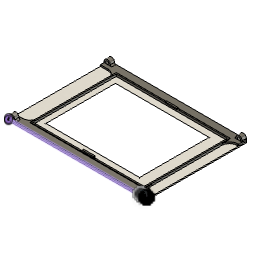
Inkplate 6 PCB Holder 130x180 mm Photo Frame v1 (Autodesk Fusion 360 design; units mm, degrees)
Autodesk Fusion 360 part; units mm, degrees
sketch "Sketch1" plane through (0, 0, 0) normal (0, 1, 0) x (1, 0, 0)
  line L0 (-90, -65) -> (90, -65)
  line L1 (90, -65) -> (90, 65)
  line L2 (90, 65) -> (-90, 65)
  line L3 (-90, 65) -> (-90, -65)
  line L4 (-90, -65) -> (90, 65) construction
  line L5 (90, -65) -> (-90, 65) construction
  line L6 (-61, -45.3) -> (61, -45.3)
  line L7 (61, -45.3) -> (61, 45.3)
  line L8 (61, 45.3) -> (-61, 45.3)
  line L9 (-61, 45.3) -> (-61, -45.3)
  line L10 (-61, -45.3) -> (61, 45.3) construction
  line L11 (61, -45.3) -> (-61, 45.3) construction
  line L12 (76.5, -45.3) -> (76.5, 45.3) construction
  line L13 (61, 53.3) -> (-61, 53.3) construction
  line L14 (-61, -54.8) -> (61, -54.8) construction
  line L15 (-68, 45.3) -> (-68, -45.3) construction
  line L16 (-68, 53.3) -> (76.5, 53.3)
  line L17 (76.5, 53.3) -> (76.5, -54.8)
  line L18 (76.5, -54.8) -> (-68, -54.8)
  line L19 (-68, -54.8) -> (-68, 53.3)
  line L20 (32.0539, 9.3491) -> (-36.4423, 9.3491) construction
  line L21 (-36.4423, 9.3491) -> (-36.4423, 14.8822) construction
  line L22 (-36.4423, 14.8822) -> (32.0539, 14.8822) construction
  line L23 (32.0539, 14.8822) -> (32.0539, 9.3491) construction
  dimension "d1" = 180
  dimension "d2" = 130
  dimension "d3" = 122
  dimension "d4" = 90.6
  dimension "d9" = 10
  dimension "d12" = 108.1
  dimension "d13" = 144.5
  constraint perpendicular L0 L1
  constraint parallel L0 L2
  constraint parallel L1 L3
  constraint coincident L4 origin
  constraint coincident L5 origin
  constraint perpendicular L6 L7
  constraint parallel L6 L8
  constraint parallel L7 L9
  constraint coincident L10 origin
  constraint coincident L11 origin
  constraint collinear L14 L18
  constraint collinear L13 L16
  constraint collinear L15 L19
  constraint collinear L12 L17
  measures "d1" distance of L1.end L2.end
  measures "d2" distance of L0.end L1.end
  measures "d3" distance of L7.end L8.end
  measures "d4" distance of L6.end L7.end
  measures "d12" distance of L16.start L18.end
  measures "d13" distance of L16.start L16.end
extrude "Extrude5" add sketch "Sketch1" along normal blind 1.5 contours L0 L1 L2 L3 | L16 L17 L18 L19 makes body 1
sketch "Sketch8" plane through (0, 1.5, 0) normal (0, 1, 0) x (-1, 0, 0)
  line L0 (61, 45.3) -> (61, -45.3)
  line L1 (61, -45.3) -> (-61, -45.3)
  line L2 (-61, -45.3) -> (-61, 45.3)
  line L3 (-61, 45.3) -> (61, 45.3)
  line L4 (90, -65) -> (90, 65)
  line L5 (90, 65) -> (-90, 65)
  line L6 (-90, 65) -> (-90, -65)
  line L7 (-90, -65) -> (90, -65)
  line L8 (68, 54.8) -> (68, -53.3)
  line L9 (-76.5, 54.8) -> (68, 54.8)
  line L10 (-61, 45.3) -> (-61, -45.3)
  line L11 (-61, -45.3) -> (61, -45.3)
  line L12 (61, -45.3) -> (61, 45.3)
  line L13 (61, 45.3) -> (-61, 45.3)
  line L14 (-76.5, -53.3) -> (-76.5, 54.8)
  line L15 (68, -53.3) -> (-76.5, -53.3)
  line L16 (-76.8, -53.6) -> (-76.8, 55.1)
  line L17 (-76.8, 55.1) -> (68.3, 55.1)
  line L18 (68.3, 55.1) -> (68.3, -53.6)
  line L19 (68.3, -53.6) -> (-76.8, -53.6)
  line L20 (-78.47, -55.27) -> (-78.47, 56.77)
  line L21 (-78.47, 56.77) -> (69.97, 56.77)
  line L22 (69.97, 56.77) -> (69.97, -55.27)
  line L23 (69.97, -55.27) -> (-78.47, -55.27)
  dimension "PCBToleranceOffset" = -0.3
extrude "Extrude1" add sketch "Sketch8" along normal blind 2.8 separate body contours L20 L21 L22 L23 makes body 2 in component "pcbHolder"
chamfer "Chamfer2" distance 1.5 angle 45 4 edges at (0, 0, 45.3) (-61, 0, 0) (61, 0, 0) (0, 0, -45.3) on bodies 1
sketch "Sketch9" plane through (0, 0, 65) normal (0, 0, 1) x (1, 0, 0)
  line L0 (-90, 0) -> (90, 0)
  line L1 (90, 0) -> (90, 1.5)
  line L2 (90, 1.5) -> (-90, 1.5)
  line L3 (-90, 1.5) -> (-90, 0)
  line L4 (-69.97, 1.5) -> (78.47, 1.5)
  line L5 (78.47, 1.5) -> (78.47, 4.3)
  line L6 (78.47, 4.3) -> (-69.97, 4.3)
  line L7 (-69.97, 4.3) -> (-69.97, 1.5)
  line L8 (78.47, 1.5) -> (90, 1.5) construction
  line L9 (84.235, 1.5) -> (84.235, 3.45) construction
  circle A0 centre (84.2347, 5.1) radius 1.65
  dimension "d145" = 1.95
  dimension "d146" = 3.3
  dimension "d147" = 3.45
  constraint coincident L4.end L5.start
  constraint coincident L1.end L2.start
  constraint midpoint L8 L9.start
  constraint perpendicular L2 L9
  constraint coincident L9.end A0
  measures "d145" distance of L9.start L9.end
  measures "d146" diameter of A0
  measures "d147" distance of L0 L9.end
sketch "Sketch1 (2)" plane through (0, 1.5, 0) normal (0, 1, 0) x (-1, 0, 0) in component "pcbHolder"
  line L0 (61, 45.3) -> (61, -45.3)
  line L1 (61, -45.3) -> (-61, -45.3)
  line L2 (-61, -45.3) -> (-61, 45.3)
  line L3 (-61, 45.3) -> (61, 45.3)
  line L4 (90, -65) -> (90, 65)
  line L5 (90, 65) -> (-90, 65)
  line L6 (-90, 65) -> (-90, -65)
  line L7 (-90, -65) -> (90, -65)
  line L8 (68.3, 55.1) -> (68.3, -53.6)
  line L9 (68.3, -53.6) -> (-76.8, -53.6)
  line L10 (-76.8, -53.6) -> (-76.8, 55.1)
  line L11 (-76.8, 55.1) -> (68.3, 55.1)
  line L12 (69.97, -55.27) -> (69.97, 56.77)
  line L13 (69.97, 56.77) -> (-78.47, 56.77)
  line L14 (-78.47, 56.77) -> (-78.47, -55.27)
  line L15 (-78.47, -55.27) -> (69.97, -55.27)
  line L16 (-78.47, 56.77) -> (-90, 56.77)
  line L17 (-90, 56.77) -> (90, 56.77)
  line L18 (90, -54.6) -> (-90, -54.6)
  constraint coincident L13.end L14.start
  constraint coincident L6 L16.end
  constraint perpendicular L6 L16
  constraint coincident L4 L17.end
  constraint perpendicular L4 L17
  constraint coincident L4 L18.start
  constraint coincident L6 L18.end
  constraint perpendicular L6 L18
extrude "Extrude2" add sketch "Sketch1 (2)" along normal blind 1.95 contours L4 L6 L7 L12 L14 L15 L18 | L4 L5 L6 L13 L16 L17 | L12 L14 L15 L18 bodies 2 in component "pcbHolder"
sketch "Sketch2" plane through (0, 1.5, 0) normal (0, 1, 0) x (-1, 0, 0) in component "pcbHolder"
  line L0 (61, 45.3) -> (61, -45.3)
  line L1 (61, -45.3) -> (-61, -45.3)
  line L2 (-61, -45.3) -> (-61, 45.3)
  line L3 (-61, 45.3) -> (61, 45.3)
  line L4 (90, -65) -> (90, 65)
  line L5 (90, 65) -> (-90, 65)
  line L6 (-90, 65) -> (-90, -65)
  line L7 (-90, -65) -> (90, -65)
  line L8 (90, -54.6) -> (69.97, -54.6)
  line L9 (90, -65) -> (90, -54.6)
  line L10 (-90, -65) -> (90, -65)
  line L11 (-90, -54.6) -> (-90, -65)
  line L12 (-78.47, -54.6) -> (-90, -54.6)
  line L13 (69.97, 56.77) -> (90, 56.77)
  line L14 (-90, 65) -> (-90, 56.77)
  line L15 (90, 65) -> (-90, 65)
  line L16 (90, 56.77) -> (90, 65)
  line L17 (-90, 56.77) -> (-78.47, 56.77)
  line L18 (-76.8, 55.1) -> (68.3, 55.1)
  line L19 (-76.8, -53.6) -> (-76.8, 55.1)
  line L20 (68.3, -53.6) -> (-76.8, -53.6)
  line L21 (68.3, 55.1) -> (68.3, -53.6)
  line L22 (-78.47, -54.6) -> (-78.47, 56.77)
  line L23 (69.97, 56.77) -> (69.97, -54.6)
  circle A0 centre (79.97, -44.6) radius 10
  circle A1 centre (-88.47, -44.6) radius 10
  circle A2 centre (79.97, 46.77) radius 10
  circle A3 centre (-88.47, 46.77) radius 10
  dimension "d150" = 10
  dimension "d151" = 10
  dimension "d152" = 10
  dimension "d153" = 10
  constraint tangent L8 A0
  constraint tangent L23 A0
  constraint tangent L12 A1
  constraint tangent L22 A1
  constraint tangent L23 A2
  constraint tangent L13 A2
  constraint tangent L17 A3
  constraint tangent L22 A3
  measures "d150" radius of A0
  measures "d151" radius of A1
  measures "d152" radius of A2
  measures "d153" radius of A3
extrude "Extrude3" add sketch "Sketch2" along normal up to surface (1.95 mm away) contours L8 L23 A0 | L13 L23 A2 | L12 L22 A1 | L17 L22 A3 bodies 2 in component "pcbHolder"
sketch "Sketch3" plane through (0, 4.3, 0) normal (0, 1, 0) x (-1, 0, 0) in component "pcbHolder"
  line L0 (68.3, 55.1) -> (68.3, -53.6)
  line L1 (68.3, -53.6) -> (-76.8, -53.6)
  line L2 (-76.8, -53.6) -> (-76.8, 55.1)
  line L3 (-76.8, 55.1) -> (68.3, 55.1)
  line L4 (69.97, -55.27) -> (69.97, 56.77)
  line L5 (69.97, 56.77) -> (-78.47, 56.77)
  line L6 (-78.47, 56.77) -> (-78.47, -55.27)
  line L7 (-78.47, -55.27) -> (69.97, -55.27)
  line L8 (-4.25, 55.1) -> (-4.25, -53.6) construction
  line L9 (-11.75, 56.1) -> (3.25, 56.1)
  line L10 (3.25, 56.1) -> (3.25, 54.1)
  line L11 (3.25, 54.1) -> (-11.75, 54.1)
  line L12 (-11.75, 54.1) -> (-11.75, 56.1)
  line L13 (-11.75, 56.1) -> (3.25, 54.1) construction
  line L14 (3.25, 56.1) -> (-11.75, 54.1) construction
  point P0 (-4.25, 55.1)
  dimension "d156" = 15
  constraint midpoint L3 P0
  constraint midpoint L1 L8.end
  constraint horizontal L9
  constraint perpendicular L9 L10
  constraint parallel L9 L11
  constraint parallel L10 L12
  constraint coincident L13 P0
  constraint coincident L14 P0
  constraint coincident P0 L8.start
  measures "d156" distance of L10.end L11.end
extrude "Extrude4" add sketch "Sketch3" along normal blind 1.5 contours L3 L10 L11 L12 | L3 L9 L10 L12 bodies 2 in component "pcbHolder"
fillet "Fillet1" radius 2 2 edges at (-3.25, 4.3, 55.6) (11.75, 4.3, 55.6) on bodies 2 in component "pcbHolder"
ref_plane "WorkPlane1" through (4.25, 2.9, 0.75) normal (0, 0, 1) x (1, 0, 0) in component "pcbHolder"
mirror "Mirror1" about plane through (4.25, 2.9, 0.75) normal (0, 0, 1) of "Extrude4", "Fillet1" in component "pcbHolder"
sketch "Sketch5" plane through (0, 0, 65) normal (0, 0, 1) x (1, 0, 0) in component "pcbHolder"
  line L0 (-90, 1.5) -> (90, 1.5)
  line L1 (90, 1.5) -> (90, 3.45)
  line L2 (90, 3.45) -> (-90, 3.45)
  line L3 (-90, 3.45) -> (-90, 1.5)
  line L4 (90, 3.45) -> (86, 3.45) construction
  line L5 (-90, 0) -> (90, 0)
  line L6 (90, 0) -> (90, 1.5)
  line L7 (90, 1.5) -> (-90, 1.5)
  line L8 (-90, 1.5) -> (-90, 0)
  circle A0 centre (86, 5.1) radius 2
  circle A1 centre (86, 5.1) radius 4
  line L9 (89.9983, 4.9837) -> (90, 3.45)
  line L10 (82.0021, 4.9715) -> (82.0021, 3.45)
  dimension "d163" = 4
  dimension "d164" = 1.95
  dimension "ScrewDiameter" = 4
  dimension "d166" = 2
  constraint coincident L1.end L2.start
  constraint perpendicular L1 L4
  constraint coincident A1 L9.start
  constraint coincident A1 L10.start
  constraint coincident L2 L10.end
  constraint perpendicular L2 L10
  measures "d163" distance of L1.end L4.end
  measures "d164" distance of L0.end L1.end
  measures "ScrewDiameter" diameter of A0
  measures "d166" distance of A0
extrude "Extrude5'" add sketch "Sketch5" against normal blind 5.5 contours L2 A0 A1 | L2 A1 L10 | L2 A1 L9 bodies 2 in component "pcbHolder"
mirror "Mirror2" about plane through (0, 0, 0) normal (1, 0, 0) of "Extrude5'" in component "pcbHolder"
mirror "Mirror3" about plane through (0, 0, 0) normal (0, 0, 1) of "Extrude5'", "Mirror2" in component "pcbHolder"
fillet "Fillet2" radius 2 4 edges at (-82.0021, 3.45, -62.25) (-82.0021, 3.45, 62.25) (82.0021, 3.45, 62.25) (82.0021, 3.45, -62.25) on bodies 2 in component "pcbHolder"
extrude "Extrude6" cut sketch "Sketch5" against normal up to surface (5.5 mm away) contours L2 A0 picked at (86.3002, 3.4048) bodies 2 in component "pcbHolder"
mirror "Mirror4" about plane through (0, 0, 0) normal (1, 0, 0) of "Extrude6" in component "pcbHolder"
mirror "Mirror5" about plane through (0, 0, 0) normal (0, 0, 1) of "Extrude6", "Mirror4" in component "pcbHolder"
sketch "Sketch4" plane through (0, 0, 65) normal (0, 0, 1) x (1, 0, 0) in component "pcbHolder"
  arc A0 (11.75, 5.8) -> (13.6865, 4.3) centre (13.6865, 6.3) ccw
  arc A1 (-5.1865, 4.3) -> (-3.25, 5.8) centre (-5.1865, 6.3) ccw
  line L0 (-3.25, 5.8) -> (11.75, 5.8)
  line L1 (77.8, 4.3) -> (13.6865, 4.3)
  line L2 (-5.1865, 4.3) -> (-69.3, 4.3)
  line L3 (77.8, 3.45) -> (77.8, 4.3)
  line L4 (-69.3, 3.45) -> (-69.3, 4.3)
  line L5 (-90, 1.5) -> (-90, 3.45)
  line L6 (90, 1.5) -> (-90, 1.5)
  line L7 (90, 3.45) -> (77.8, 3.45)
  line L8 (-69.3, 3.45) -> (-90, 3.45)
  line L9 (90, 1.5) -> (90, 3.45)
extrude "Extrude1'" [suppressed]
extrude "Extrude2'" [suppressed]
chamfer "Chamfer1" [suppressed]
sketch "Sketch2 (2)" plane through (0, 3.3, 0) normal (0, 1, 0) x (-1, 0, 0)
  line L0 (-76.5, 54.8) -> (68, 54.8)
  line L1 (68, 54.8) -> (68, -53.3)
  line L2 (68, -53.3) -> (-76.5, -53.3)
  line L3 (-76.5, -53.3) -> (-76.5, 54.8)
  line L4 (90, -65) -> (90, 65)
  line L5 (90, 65) -> (-90, 65)
  line L6 (-90, 65) -> (-90, -65)
  line L7 (-90, -65) -> (90, -65)
  line L8 (-78, -54.8) -> (-78, 56.3)
  line L9 (-78, 56.3) -> (69.5, 56.3)
  line L10 (69.5, 56.3) -> (69.5, -54.8)
  line L11 (69.5, -54.8) -> (-78, -54.8)
  dimension "d20" = -1.5
extrude "Extrude3'" [suppressed]
sketch "Sketch3 (2)" plane through (0, 3.3, 0) normal (0, 1, 0) x (-1, 0, 0)
  line L0 (69.5, -54.8) -> (-78, -54.8)
  line L1 (-78, -54.8) -> (-78, 56.3)
  line L2 (-78, 56.3) -> (69.5, 56.3)
  line L3 (69.5, 56.3) -> (69.5, -54.8)
  line L4 (90, -65) -> (90, 65)
  line L5 (90, 65) -> (-90, 65)
  line L6 (-90, 65) -> (-90, -65)
  line L7 (-90, -65) -> (90, -65)
copy_body "Body->Comp1" [suppressed] in component "Component"
ref_plane "WorkPlane2" through (0, 1.65, 62) normal (0, 0, 1) x (1, 0, 0)
sketch "Sketch4 (2)" plane through (0, 0, 62) normal (0, 0, 1) x (1, 0, 0)
  line L0 (-90, 0) -> (90, 0)
  line L1 (90, 0) -> (90, 3.3)
  line L2 (90, 3.3) -> (-90, 3.3)
  line L3 (-90, 3.3) -> (-90, 0)
  line L4 (-68, 0.55) -> (76.5, 0.55)
  line L5 (76.5, 0.55) -> (76.5, 4.3)
  line L6 (76.5, 4.3) -> (-68, 4.3)
  line L7 (-68, 4.3) -> (-68, 0.55)
  line L8 (82.5, -5.45) -> (82.5, 10.3) construction
  line L9 (82.5, 10.3) -> (-74, 10.3) construction
  line L10 (-74, 10.3) -> (-74, -5.45) construction
  line L11 (-74, -5.45) -> (82.5, -5.45) construction
  line L12 (-74, 3.3) -> (-74, 5.1) construction
  circle A0 centre (-74, 5.1) radius 1.65
  line L13 (4.25, -5.45) -> (4.25, 10.3)
  circle A1 centre (-74, 5.1) radius 4
  circle A2 centre (82.5, 5.1) radius 4
  dimension "d85" = 6
  dimension "d86" = 1.8
  dimension "d87" = 3.3
  dimension "d88" = 8
  constraint coincident L10 L12.start
  constraint coincident L2 L12.start
  constraint perpendicular L2 L12
  constraint coincident L12.end A0.centre
  constraint midpoint L11 L13.start
  constraint midpoint L9 L13.end
  constraint symmetric L13 A1 A2
  measures "d86" distance of L12.start L12.end
  measures "d87" diameter of A0
  measures "d88" diameter of A1
extrude "Extrude4'" [suppressed]
extrude "Extrude8" [no effect] in component "Component"
ref_plane "WorkPlane3" through (0, 1.65, 0) normal (0, 0, -1) x (-1, 0, 0)
mirror "Mirror1'" [suppressed]
mirror "Mirror1''" [no effect] in component "Component"
sketch "Sketch5 (2)" plane through (0, 3.3, 0) normal (0, 1, 0) x (-1, 0, 0)
  line L0 (70.4279, -62) -> (70.4279, -37)
  line L1 (70.4279, -37) -> (77.5721, -37)
  line L2 (77.5721, -37) -> (77.5721, -62)
  line L3 (77.5721, -62) -> (70.4279, -62)
  line L4 (-86.0721, -62) -> (-86.0721, -37)
  line L5 (-86.0721, -37) -> (-78.9279, -37)
  line L6 (-78.9279, -37) -> (-78.9279, -62)
  line L7 (-78.9279, -62) -> (-86.0721, -62)
  line L8 (70.4279, 37) -> (70.4279, 62)
  line L9 (70.4279, 62) -> (77.5721, 62)
  line L10 (77.5721, 62) -> (77.5721, 37)
  line L11 (77.5721, 37) -> (70.4279, 37)
  line L12 (-86.0721, 37) -> (-86.0721, 62)
  line L13 (-86.0721, 62) -> (-78.9279, 62)
  line L14 (-78.9279, 62) -> (-78.9279, 37)
  line L15 (-78.9279, 37) -> (-86.0721, 37)
  line L16 (69.5, -54.8) -> (-78, -54.8)
  line L17 (-78, -54.8) -> (-78, 56.3)
  line L18 (-78, 56.3) -> (69.5, 56.3)
  line L19 (69.5, 56.3) -> (69.5, -54.8)
  line L20 (90, -65) -> (90, 65)
  line L21 (90, 65) -> (-90, 65)
  line L22 (-90, 65) -> (-90, -65)
  line L23 (-90, -65) -> (90, -65)
  line L24 (-90, 0) -> (90, 0)
  line L25 (88, 63) -> (-88, 63) construction
  line L26 (-88, 63) -> (-88, -63) construction
  line L27 (-88, -63) -> (88, -63) construction
  line L28 (88, -63) -> (88, 63) construction
  line L29 (85.5, 60.5) -> (-85.5, 60.5) construction
  line L30 (-85.5, 60.5) -> (-85.5, -60.5) construction
  line L31 (-85.5, -60.5) -> (85.5, -60.5) construction
  line L32 (85.5, -60.5) -> (85.5, 60.5) construction
  line L33 (83.5, 58.5) -> (-83.5, 58.5)
  line L34 (-83.5, 58.5) -> (-83.5, -58.5)
  line L35 (-83.5, -58.5) -> (83.5, -58.5)
  line L36 (83.5, -58.5) -> (83.5, 58.5)
  line L37 (77.5721, -60.5) -> (70.4279, -60.5)
  line L38 (70.4279, -60.5) -> (70.4279, -65)
  line L39 (70.4279, -65) -> (77.5721, -65)
  line L40 (77.5721, -65) -> (77.5721, -60.5)
  line L41 (77.5721, -58.5) -> (70.4279, -58.5)
  line L42 (70.4279, -58.5) -> (70.4279, -60.5)
  line L43 (70.4279, -60.5) -> (77.5721, -60.5)
  line L44 (77.5721, -60.5) -> (77.5721, -58.5)
  line L45 (77.5721, -62) -> (70.4279, -62)
  line L46 (70.4279, -62) -> (70.4279, -60.5)
  line L47 (70.4279, -60.5) -> (77.5721, -60.5)
  line L48 (77.5721, -60.5) -> (77.5721, -62)
  line L49 (70.4279, -58.5) -> (68.4279, -58.5) construction
  line L50 (68.4279, -58.5) -> (70.4279, -58.5)
  line L51 (70.4279, -58.5) -> (70.4279, -65)
  line L52 (70.4279, -65) -> (68.4279, -65)
  line L53 (68.4279, -65) -> (68.4279, -58.5)
  line L54 (74, -65) -> (74, -37)
  line L55 (79.5721, -65) -> (79.5721, -58.5)
  line L56 (77.5721, -63) -> (70.4279, -63)
  line L57 (70.4279, -63) -> (70.4279, -60.5)
  line L58 (70.4279, -60.5) -> (77.5721, -60.5)
  line L59 (77.5721, -60.5) -> (77.5721, -63)
  dimension "d99" = -2
  dimension "d101" = -4.5
  dimension "d102" = -6.5
  dimension "d103" = 2
  dimension "d136" = 7.1442
  constraint midpoint L22 L24.start
  constraint midpoint L20 L24.end
  constraint horizontal L37
  constraint vertical L38
  constraint horizontal L39
  constraint vertical L40
  constraint coincident L23 L38.end
  constraint coincident L2 L37.start
  constraint coincident L31 L37.start
  constraint horizontal L41
  constraint vertical L42
  constraint horizontal L43
  constraint vertical L44
  constraint coincident L2 L41.start
  constraint coincident L35 L41.start
  constraint horizontal L45
  constraint vertical L46
  constraint horizontal L47
  constraint vertical L48
  constraint coincident L2.end L3.start
  constraint collinear L0 L38
  constraint perpendicular L42 L49
  constraint horizontal L50
  constraint vertical L51
  constraint horizontal L52
  constraint vertical L53
  constraint midpoint L39 L54.start
  constraint midpoint L1 L54.end
  constraint symmetric L49.end L54 L55.end
  constraint symmetric L52.end L54 L55.start
  constraint horizontal L56
  constraint vertical L57
  constraint horizontal L58
  constraint vertical L59
  constraint coincident L40 L56.start
  constraint coincident L27 L56.start
  measures "d103" distance of L41.end L49.end
  measures "d136" distance of L2.end L0.start
extrude "Extrude9" [suppressed] in component "Component"
fillet "Fillet1'" [suppressed] in component "Component"
ref_plane "WorkPlane4" through (4.25, 3.8, 0.75) normal (-1, 0, 0) x (0, 0, 1)
mirror "Mirror2'" [suppressed] in component "Component"
mirror "Mirror3'" [suppressed] in component "Component"
mirror "Mirror4'" [suppressed] in component "Component"
fillet "Fillet2'" [suppressed] in component "Component"
fillet "Fillet3" [suppressed] in component "Component"
extrude "Extrude12" [suppressed] in component "Component"
fillet "Fillet4" [suppressed] in component "Component"
extrude "Extrude10" [suppressed] in component "Component"
mirror "Mirror5'" [suppressed] in component "Component"
sketch "Sketch6" plane through (0, 8.3, 0) normal (0, 1, 0) x (-1, 0, 0)
  line L0 (70.4279, -63) -> (70.4279, -60.5)
  line L1 (70.4279, -60.5) -> (77.5721, -60.5)
  line L2 (77.5721, -60.5) -> (77.5721, -63)
  line L3 (69.928, -65) -> (78.072, -65)
  line L4 (78.072, -58.5) -> (69.928, -58.5)
  line L5 (70.4279, 60.5) -> (70.4279, 63)
  line L6 (77.5721, 63) -> (77.5721, 60.5)
  line L7 (77.5721, 60.5) -> (70.4279, 60.5)
  line L8 (78.072, 65) -> (69.928, 65)
  line L9 (69.928, 58.5) -> (78.072, 58.5)
  line L10 (-78.9279, -60.5) -> (-78.9279, -63)
  line L11 (-86.0721, -63) -> (-86.0721, -60.5)
  line L12 (-86.0721, -60.5) -> (-78.9279, -60.5)
  line L13 (-88, -65) -> (-76.9279, -65)
  line L14 (-76.9279, -58.5) -> (-90, -58.5)
  line L15 (-78.9279, 63) -> (-78.9279, 60.5)
  line L16 (-78.9279, 60.5) -> (-86.0721, 60.5)
  line L17 (-86.0721, 60.5) -> (-86.0721, 63)
  line L18 (-76.9279, 65) -> (-88, 65)
  line L19 (-90, 58.5) -> (-76.9279, 58.5)
  line L20 (77.5721, -63) -> (70.4279, -63)
  line L21 (70.4279, 63) -> (77.5721, 63)
  line L22 (-78.9279, -63) -> (-86.0721, -63)
  line L23 (-86.0721, 63) -> (-78.9279, 63)
  line L24 (78.072, -65) -> (78.072, -58.5)
  line L25 (69.928, -58.5) -> (69.928, -65)
  line L26 (78.072, 58.5) -> (78.072, 65)
  line L27 (69.928, 65) -> (69.928, 58.5)
  arc A0 (-90, -63) -> (-88, -65) centre (-88, -63) ccw
  line L28 (-76.9279, -65) -> (-76.9279, -58.5)
  line L29 (-90, -58.5) -> (-90, -63)
  arc A1 (-88, 65) -> (-90, 63) centre (-88, 63) ccw
  line L30 (-90, 63) -> (-90, 58.5)
  line L31 (-76.9279, 58.5) -> (-76.9279, 65)
extrude "Extrude11" [suppressed] in component "Component"
fillet "Fillet5" [suppressed] in component "Component"
ref_plane "WorkPlane5" through (0, 1.5, 0) normal (0, -1, 0) x (-1, 0, 0)
split "Split1" [suppressed] in component "Component"
sketch "Sketch7" plane through (0, 3.3, 0) normal (0, 1, 0) x (-1, 0, 0)
  arc A0 (88, -65) -> (90, -63) centre (88, -63) ccw
  line L0 (90, -63) -> (90, 63)
  arc A1 (90, 63) -> (88, 65) centre (88, 63) ccw
  line L1 (88, 65) -> (85.4882, 65)
  line L2 (85.4882, 65) -> (85.4882, 58.5)
  line L3 (85.4882, 58.5) -> (77.5721, 58.5)
  line L4 (77.5721, 58.5) -> (77.5721, 37)
  line L5 (77.5721, 37) -> (70.4279, 37)
  line L6 (70.4279, 37) -> (70.4279, 58.5)
  line L7 (70.4279, 58.5) -> (62.5118, 58.5)
  line L8 (62.5118, 58.5) -> (62.5118, 65)
  line L9 (62.5118, 65) -> (-71.0118, 65)
  line L10 (-71.0118, 65) -> (-71.0118, 58.5)
  line L11 (-71.0118, 58.5) -> (-78.9279, 58.5)
  line L12 (-78.9279, 58.5) -> (-78.9279, 37)
  line L13 (-78.9279, 37) -> (-86.0721, 37)
  line L14 (-86.0721, 37) -> (-86.0721, 58.5)
  line L15 (-86.0721, 58.5) -> (-90, 58.5)
  line L16 (-90, 58.5) -> (-90, -58.5)
  line L17 (-90, -58.5) -> (-86.0721, -58.5)
  line L18 (-86.0721, -58.5) -> (-86.0721, -37)
  line L19 (-86.0721, -37) -> (-78.9279, -37)
  line L20 (-78.9279, -37) -> (-78.9279, -58.5)
  line L21 (-78.9279, -58.5) -> (-71.0118, -58.5)
  line L22 (-71.0118, -58.5) -> (-71.0118, -65)
  line L23 (-71.0118, -65) -> (62.5118, -65)
  line L24 (62.5118, -65) -> (62.5118, -58.5)
  line L25 (62.5118, -58.5) -> (70.4279, -58.5)
  line L26 (70.4279, -58.5) -> (70.4279, -37)
  line L27 (70.4279, -37) -> (77.5721, -37)
  line L28 (77.5721, -37) -> (77.5721, -58.5)
  line L29 (77.5721, -58.5) -> (85.4882, -58.5)
  line L30 (85.4882, -58.5) -> (85.4882, -65)
  line L31 (85.4882, -65) -> (88, -65)
  line L32 (69.5, -54.8) -> (-78, -54.8)
  line L33 (-78, -54.8) -> (-78, 56.3)
  line L34 (-78, 56.3) -> (69.5, 56.3)
  line L35 (69.5, 56.3) -> (69.5, -54.8)
  line L36 (69.5, -58.5) -> (90, -58.5)
  line L37 (90, -58.5) -> (90, 58.5)
  line L38 (90, 58.5) -> (69.5, 58.5)
  line L39 (69.5, 58.5) -> (69.5, -58.5)
  line L40 (-78, -58.5) -> (-90, -58.5)
  line L41 (-90, -58.5) -> (-90, 58.5)
  line L42 (-90, 58.5) -> (-78, 58.5)
  line L43 (-78, 58.5) -> (-78, -58.5)
  constraint horizontal L36
  constraint vertical L37
  constraint horizontal L38
  constraint vertical L39
  constraint coincident L0 L37.end
  constraint coincident L25 L36.start
  constraint horizontal L40
  constraint vertical L41
  constraint horizontal L42
  constraint vertical L43
  constraint coincident L15.end L16.start
  constraint coincident L21 L40.start
extrude "Extrude13" [suppressed] in component "Component"
component "pcbHolder" placed x (1, 0, 0) y (0, 1, 0) z (0, 0, 1) at (0, 0, 0)
equation "ClipFullExtensionLength = 5 mm"
equation "ClipExtensionTipWidth = 3 mm"
equation "ClipBodyWidth = 10 mm"
equation "ClipBodyLength = 8 mm"
equation "ClipThickness = 1.5 mm"
equation "ClipToleranceWidth = 0.2 mm"
equation "d86 = ( 3.0 / 2 ) * 1 mm + 0.3 mm"
equation "d87 = 3.00 mm + 0.3 mm"
equation "NutThickness = 2.5 mm"
equation "d101 = -( 2 mm + NutThickness )"
equation "d102 = -( 2 mm + 2 mm + NutThickness )"
equation "PCBWallThickness = 1.67 mm"
equation "d141 = -PCBWallThickness + PCBToleranceOffset"
equation "PCBWallHeight = 2.8 mm"
equation "d163 = 2 mm + ( 4 / 2 ) * 1 mm"
named bodies: "passepartout", "PCB holder v1"
